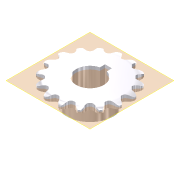
# Autodesk Inventor part: 25 sprocket 16T 500Key
Saved by Autodesk Inventor 2011 (Build 150239000, 239)
## iProperties
Created: 2012-05-18
Part Number: 25 sprocket 16T 500Key
Material: Aluminum-6061
Document SubType Name: Modeling
Designer: niemitalo_dan
Mass: 9.8579 g
Surface Area: 27.0741 cm^2
Volume: 3.6376 cm^3
Density: 2.71 g/cm^3
CustomPartVersion: 1
Author: niemitalo_dan
Title: 25 sprocket 16T 500Ke
Autodesk Inventor part; units mm, degrees
ref_plane "YZ Plane" through (0, 0, 0) normal (1, 0, 0) x (0, 1, 0)
ref_plane "XZ Plane" through (0, 0, 0) normal (0, 1, 0) x (-1, 0, 0)
sketch "500Key" plane through (0, 0, 0) normal (0, 0, 1) x (1, 0, 0)
  arc A0 (-1.5875, 6.1746) -> (1.5875, 6.1746) centre (0, 0) ccw
  line L0 (1.5875, 6.1746) -> (1.5875, 8.5558)
  line L1 (1.5875, 8.5558) -> (-1.5875, 8.5558)
  line L2 (-1.5875, 8.5558) -> (-1.5875, 6.1746)
  point P0 (0, 6.9242)
  dimension "d54" = 12.7508
  dimension "d55" = 3.175
  dimension "d56" = 2.3813
  measures "d54" diameter of A0
  measures "d55" distance of L0.end L1.end
  measures "d56" distance of L0.start L0.end
sketch "Theoretical Tooth Profile" plane through (0, 0, 0) normal (0, 0, 1) x (1, 0, 0)
  circle A0 centre (0, 0) radius 16.2745 construction
  line L0 (0, 0) -> (0, 16.2745) construction
  line L1 (0, 0) -> (6.228, 15.0357) construction
  circle A1 centre (0, 0) radius 17.8668
  arc A2 (-1.2997, 15.2314) -> (1.2997, 15.2314) centre (0, 16.2745) ccw
  line L2 (0, 16.2745) -> (6.228, 15.0357) construction
  line L3 (0, 16.2745) -> (2.0589, 17.927) construction
  line L4 (2.0589, 17.927) -> (-1.8676, 16.1582) construction
  arc A3 (2.9468, 17.6221) -> (2.023, 16.5031) centre (4.5312, 15.3732) ccw
  arc A4 (-2.023, 16.5031) -> (-2.9468, 17.6221) centre (-4.5312, 15.3732) ccw
  line L5 (-4.5312, 15.3732) -> (-2.023, 16.5031) construction
  arc A5 (-1.8676, 16.1582) -> (-1.2997, 15.2314) centre (2.0589, 17.927) ccw
  line L6 (-1.8676, 16.1582) -> (-2.023, 16.5031)
  arc A6 (1.2997, 15.2314) -> (1.8676, 16.1582) centre (-2.0589, 17.927) ccw
  line L7 (2.023, 16.5031) -> (1.8676, 16.1582)
  line L8 (0, 0) -> (3.4856, 17.5235) construction
  point P0 (3.114, 15.6551)
  dimension "d0" = 32.549
  dimension "d2" = 22.5
  dimension "d3" = 1.6665
  dimension "d10" = 128.75
  dimension "d11" = 14.5
  dimension "d12" = 2.64
  dimension "d13" = 4.3065
  dimension "d14" = 4.62
  dimension "d23" = 1.905
  constraints: 18 end point, 15 point on circle, 7 centre point, 3 coincident, 3 point on line, 3 symmetric about line, 3 tangent, 1 equal radius, 1 midpoint, 1 parallel, 1 vertical, 1 other
  measures "d0" diameter of A0
  measures "d2" angle of L1 L0
  measures "d3" radius of A2
  measures "d10" angle of L3 L0
  measures "d11" angle of L4 L3
  measures "d12" distance of L2.start L3.end
  measures "d13" distance of L3.end L4.end
  measures "d14" distance of A3.centre L0.end
  measures "d23" distance from line of L8.end L2
sketch "Tooth Profile" plane through (0, 0, 0) normal (0, 0, 1) x (1, 0, 0)
  circle A0 centre (0, 0) radius 17.8668 projected
  line L0 (0, 0) -> (0, 16.2745) construction
  line L1 (0, 16.2745) -> (1.5361, 15.6284) construction
  arc A1 (-1.5361, 15.6284) -> (1.5361, 15.6284) centre (0, 16.2745) ccw
  line L2 (-1.5361, 15.6284) -> (0, 16.2745) construction
  arc A2 (-1.5361, 15.6284) -> (-2.8175, 17.6432) centre (-8.1066, 12.8647) ccw
  arc A3 (2.8175, 17.6432) -> (1.5361, 15.6284) centre (8.1066, 12.8647) ccw
  dimension "d44" = 134.375
  dimension "d45" = 1.6665
  dimension "d46" = 7.128
  constraints: 8 point on circle, 7 end point, 3 centre point, 2 tangent, 1 coincident, 1 equal radius, 1 symmetric about line, 1 vertical
  measures "d44" angle of L1 L2
  measures "d45" radius of A1
  measures "d46" radius of A3
sketch "Section Profile" plane through (0, 0, 0) normal (1, 0, 0) x (0, 1, 0)
  line L0 (17.8668, 0) -> (-17.8668, 0) projected
  line L1 (8.7774, 1.4415) -> (-8.7774, 1.4415)
  line L2 (-8.7774, 1.4415) -> (-8.7774, -1.4415)
  line L3 (-8.7774, -1.4415) -> (8.7774, -1.4415)
  line L4 (8.7774, -1.4415) -> (8.7774, 1.4415)
  line L5 (8.7774, 1.4415) -> (17.8668, 1.4415) construction
  line L6 (17.8668, 1.4415) -> (17.8668, -1.4415) construction
  line L7 (17.8668, -1.4415) -> (8.7774, -1.4415) construction
  line L8 (8.7774, -1.4415) -> (8.7774, 1.4415)
  arc A0 (17.8668, 0.616) -> (14.7359, 1.4415) centre (14.7359, -4.9085) ccw
  arc A1 (14.7359, -1.4415) -> (17.8668, -0.616) centre (14.7359, 4.9085) ccw
  line L9 (14.7359, 1.4415) -> (0, 1.4415)
  line L10 (0, 1.4415) -> (0, -1.4415)
  line L11 (0, -1.4415) -> (14.7359, -1.4415)
  line L12 (0, 1.4415) -> (0, -1.4415)
  line L13 (17.8668, 0.616) -> (17.8668, -0.616)
  point P0 (0, 0)
  point P1 (0, 0)
  dimension "d30" = 2.883
  dimension "d31" = 17.5548
  dimension "d32" = 2.883
  dimension "d33" = 0.8255
  dimension "d34" = 6.35
  dimension "d43" = 1.4415
  constraints: 26 end point, 7 midpoint, 5 perpendicular, 4 parallel, 4 point on circle, 3 point on line, 3 symmetric about line, 2 centre point, 2 horizontal, 2 tangent, 1 collinear, 1 other
  measures "d30" distance between parallel lines of L7 L5
  measures "d31" distance between parallel lines of L2 L4
  measures "d32" distance between parallel lines of L3 L1
  measures "d33" distance from line of L13.start L5
  measures "d34" radius of A0
  measures "d43" distance between parallel lines of L3 L0
revolve "Shroud" add sketch "Section Profile" angle 360 about axis through (0, 0, 1.4415) along (0, 0, -1) contours L10 L3 L2 L0 | L0 L2 L1 L10
revolve "Strand" add sketch "Section Profile" angle 360 about axis through (0, 0, 1.4415) along (0, 0, -1) contours L13 A1 L11 L4 L0 | L0 L4 L9 A0 L13 | L4 L3 L10 L0 | L0 L10 L1 L4
pattern_of_one "Strand Pattern"
extrude "Theoretical Tooth" cut sketch "Theoretical Tooth Profile" along normal through all both and the other way through all contours A3 L7 A6 A2 A5 L6 A4 A1 picked at (0.3288, 16.1008)
extrude "Tooth" [suppressed]
pattern_circular "Tooth Pattern" count 16 over 360 about axis through (0, 0, -10) along (0, 0, 1) of "Theoretical Tooth"
ref_plane "Timing Plane" through (0, 16.2745, 0) normal (1, 0, 0) x (0, 1, 0)
sketch "Sketch4" plane through (0, 16.2745, -1.4415) normal (0, 0, -1) x (-1, 0, 0)
  arc A0 (-0.6091, -1.5512) -> (-5.0716, -2.4388) centre (0, -16.2745) ccw projected
  circle A1 centre (0, -16.2745) radius 10.795
  dimension "d51" = 21.59
  constraints: 1 centre point, 1 coincident
  measures "d51" diameter of A1
extrude "Extrusion4" add sketch "Sketch4" along normal blind 7.493
sketch "Sketch5" plane through (0, 16.2745, 1.4415) normal (0, 0, 1) x (1, 0, 0)
  arc A0 (-0.6091, -1.5512) -> (-5.0716, -2.4388) centre (0, -16.2745) ccw projected
  arc A1 (-1.5875, -10.0999) -> (1.5875, -10.0999) centre (0, -16.2745) ccw
  line L0 (1.5875, -10.0999) -> (1.5875, -7.7187)
  line L1 (1.5875, -7.7187) -> (-1.5875, -7.7187)
  line L2 (-1.5875, -7.7187) -> (-1.5875, -10.0999)
  point P0 (0, 0)
  constraints: 1 other
extrude "Extrusion5" cut sketch "Sketch5" against normal through all
sketch "Sketch6" plane through (0, 16.2745, 1.4415) normal (0, 0, 1) x (1, 0, 0)
  arc A0 (-1.5875, -10.0999) -> (1.5875, -10.0999) centre (0, -16.2745) ccw projected
  line L0 (-1.5875, -10.0999) -> (-1.5875, -7.7187) projected
  line L1 (-1.5875, -7.7187) -> (1.5875, -7.7187) projected
  line L2 (1.5875, -7.7187) -> (1.5875, -10.0999) projected
  arc A1 (5.0716, -2.4388) -> (6.1971, -2.905) centre (6.228, -1.2388) ccw projected
  arc A2 (5.0716, -2.4388) -> (0.6091, -1.5512) centre (0, -16.2745) ccw projected
  arc A3 (-0.6091, -1.5512) -> (0.6091, -1.5512) centre (0, 0) ccw projected
  arc A4 (-0.6091, -1.5512) -> (-5.0716, -2.4388) centre (0, -16.2745) ccw projected
  arc A5 (-6.1971, -2.905) -> (-5.0716, -2.4388) centre (-6.228, -1.2388) ccw projected
  arc A6 (-6.1971, -2.905) -> (-9.9802, -5.4328) centre (0, -16.2745) ccw projected
  arc A7 (-10.8417, -6.2943) -> (-9.9802, -5.4328) centre (-11.5078, -4.7667) ccw projected
  arc A8 (-10.8417, -6.2943) -> (-13.3695, -10.0774) centre (0, -16.2745) ccw projected
  arc A9 (-13.8357, -11.2029) -> (-13.3695, -10.0774) centre (-15.0357, -10.0465) ccw projected
  arc A10 (-13.8357, -11.2029) -> (-14.7233, -15.6654) centre (0, -16.2745) ccw projected
  arc A11 (-14.7233, -16.8837) -> (-14.7233, -15.6654) centre (-16.2745, -16.2745) ccw projected
  arc A12 (-14.7233, -16.8837) -> (-13.8357, -21.3461) centre (0, -16.2745) ccw projected
  arc A13 (-13.3695, -22.4717) -> (-13.8357, -21.3461) centre (-15.0357, -22.5025) ccw projected
  arc A14 (-13.3695, -22.4717) -> (-10.8417, -26.2548) centre (0, -16.2745) ccw projected
  arc A15 (-9.9802, -27.1162) -> (-10.8417, -26.2548) centre (-11.5078, -27.7823) ccw projected
  arc A16 (-9.9802, -27.1162) -> (-6.1971, -29.644) centre (0, -16.2745) ccw projected
  arc A17 (-5.0716, -30.1102) -> (-6.1971, -29.644) centre (-6.228, -31.3102) ccw projected
  arc A18 (-5.0716, -30.1102) -> (-0.6091, -30.9978) centre (0, -16.2745) ccw projected
  arc A19 (0.6091, -30.9978) -> (-0.6091, -30.9978) centre (0, -32.549) ccw projected
  arc A20 (0.6091, -30.9978) -> (5.0716, -30.1102) centre (0, -16.2745) ccw projected
  arc A21 (6.1971, -29.644) -> (5.0716, -30.1102) centre (6.228, -31.3102) ccw projected
  arc A22 (6.1971, -29.644) -> (9.9802, -27.1162) centre (0, -16.2745) ccw projected
  arc A23 (10.8417, -26.2548) -> (9.9802, -27.1162) centre (11.5078, -27.7823) ccw projected
  arc A24 (10.8417, -26.2548) -> (13.3695, -22.4717) centre (0, -16.2745) ccw projected
  arc A25 (13.8357, -21.3461) -> (13.3695, -22.4717) centre (15.0357, -22.5025) ccw projected
  arc A26 (13.8357, -21.3461) -> (14.7233, -16.8837) centre (0, -16.2745) ccw projected
  arc A27 (14.7233, -15.6654) -> (14.7233, -16.8837) centre (16.2745, -16.2745) ccw projected
  arc A28 (14.7233, -15.6654) -> (13.8357, -11.2029) centre (0, -16.2745) ccw projected
  arc A29 (13.3695, -10.0774) -> (13.8357, -11.2029) centre (15.0357, -10.0465) ccw projected
  arc A30 (13.3695, -10.0774) -> (10.8417, -6.2943) centre (0, -16.2745) ccw projected
  arc A31 (9.9802, -5.4328) -> (10.8417, -6.2943) centre (11.5078, -4.7667) ccw projected
  arc A32 (9.9802, -5.4328) -> (6.1971, -2.905) centre (0, -16.2745) ccw projected
  line L3 (-2, -13.2745) -> (-2, -11.6919) projected
  arc A33 (-2, -11.6919) -> (2, -11.6919) centre (0, -16.2745) ccw projected
  line L4 (2, -13.2745) -> (2, -11.6919) projected
  line L5 (-2, -13.2745) -> (2, -13.2745) projected
equation "\"d3\" = 0.5 * da_Dr + da_SC"
equation "\"d12\" = 0.8 * da_Dr"
equation "\"d13\" = 1.3 * da_Dr + da_SC"
equation "\"d14\" = 1.4 * da_Dr"
equation "\"d23\" = da_Ha"
equation "\"d44\" = da_Alfa"
equation "\"d45\" = da_Ri"
equation "\"d46\" = da_Re"
equation "\"d30\" = da_Bf"
equation "\"d31\" = da_Ds"
equation "\"d32\" = da_Bs"
equation "\"d33\" = da_Ba"
equation "\"d34\" = da_Rx"
equation "\"d40\" = da_pt"
equation "\"form_type\" = 0"
equation "\"da_p\" = 6.35"
equation "\"da_Dr\" = 3.3"
equation "\"da_SC\" = 0.0165"
equation "\"da_Ha\" = 1.905"
equation "\"da_pt\" = 6.4"
equation "\"da_Bf\" = 2.883"
equation "\"da_Ba\" = 0.8255"
equation "\"da_Rx\" = 6.35"
equation "\"da_Ra\" = 0.254"
equation "\"da_Bs\" = 2.883"
equation "\"da_Ds\" = 17.55481"
equation "\"da_Re\" = 7.128"
equation "\"da_Ri\" = 1.6665"
equation "\"da_Alfa\" = 134.375deg"
body "Solid1"
